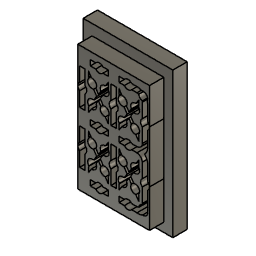
Case v4 (Autodesk Fusion 360 design; units mm, degrees)
Autodesk Fusion 360 part; units mm, degrees
note: some values were not read from the file. Set by a fixed rule: which sketch regions a step uses.
sketch "Skizze1" plane through (0, 0, 0) normal (0, 1, 0) x (1, 0, 0)
  line L0 (0, 0) -> (50, 0)
  line L1 (50, 0) -> (50, -81)
  line L2 (50, -81) -> (0, -81)
  line L3 (0, -81) -> (0, 0)
  line L4 (5, 0) -> (5, -5)
  line L5 (5, -5) -> (5, -75)
  line L6 (5, -75) -> (45, -75)
  line L7 (45, -75) -> (45, -5)
  line L8 (5, -5) -> (45, -5)
  line L9 (12, -10) -> (22, -10)
  line L10 (22, -10) -> (22, -13)
  line L11 (22, -13) -> (12, -13)
  line L12 (12, -13) -> (12, -10)
  line L13 (28, -10) -> (38, -10)
  line L14 (38, -10) -> (38, -13)
  line L15 (38, -13) -> (28, -13)
  line L16 (28, -13) -> (28, -10)
  line L17 (9, -16) -> (6, -16)
  line L18 (6, -16) -> (6, -36)
  line L19 (6, -36) -> (9, -36)
  line L20 (9, -36) -> (9, -16)
  line L21 (23.5, -16) -> (26.5, -16)
  line L22 (26.5, -16) -> (26.5, -36)
  line L23 (26.5, -36) -> (23.5, -36)
  line L24 (23.5, -36) -> (23.5, -16)
  line L25 (41, -16) -> (44, -16)
  line L26 (44, -16) -> (44, -36)
  line L27 (44, -36) -> (41, -36)
  line L28 (41, -36) -> (41, -16)
  line L29 (38, -42) -> (28, -42)
  line L30 (22, -39) -> (22, -42)
  line L31 (38, -39) -> (38, -42)
  line L32 (12, -39) -> (22, -39)
  line L33 (28, -39) -> (38, -39)
  line L34 (22, -42) -> (12, -42)
  line L35 (28, -42) -> (28, -39)
  line L36 (12, -42) -> (12, -39)
  line L37 (23.5, -45) -> (26.5, -45)
  line L38 (28, -68) -> (38, -68)
  line L39 (6, -45) -> (6, -65)
  line L40 (44, -65) -> (41, -65)
  line L41 (9, -65) -> (9, -45)
  line L42 (26.5, -45) -> (26.5, -65)
  line L43 (38, -71) -> (28, -71)
  line L44 (26.5, -65) -> (23.5, -65)
  line L45 (41, -45) -> (44, -45)
  line L46 (41, -65) -> (41, -45)
  line L47 (23.5, -65) -> (23.5, -45)
  line L48 (12, -68) -> (22, -68)
  line L49 (12, -71) -> (12, -68)
  line L50 (38, -68) -> (38, -71)
  line L51 (9, -45) -> (6, -45)
  line L52 (22, -71) -> (12, -71)
  line L53 (28, -71) -> (28, -68)
  line L54 (44, -45) -> (44, -65)
  line L55 (6, -65) -> (9, -65)
  line L56 (22, -68) -> (22, -71)
  line L57 (11, -65) -> (11, -62)
  line L58 (22, -45) -> (22, -48)
  line L59 (22, -48) -> (11, -65)
  line L60 (11, -62) -> (22, -45)
  line L61 (22, -65) -> (22, -62)
  line L62 (22, -62) -> (11, -45)
  line L63 (11, -45) -> (11, -48)
  line L64 (11, -48) -> (22, -65)
  line L65 (22, -16) -> (22, -19)
  line L66 (22, -19) -> (11, -36)
  line L67 (11, -36) -> (11, -33)
  line L68 (11, -19) -> (22, -36)
  line L69 (11, -16) -> (11, -19)
  line L70 (11, -33) -> (22, -16)
  line L71 (22, -36) -> (22, -33)
  line L72 (22, -33) -> (11, -16)
  line L73 (22, -45) -> (22, -48)
  line L74 (22, -48) -> (11, -65)
  line L75 (11, -65) -> (11, -62)
  line L76 (11, -48) -> (22, -65)
  line L77 (11, -45) -> (11, -48)
  line L78 (11, -62) -> (22, -45)
  line L79 (22, -65) -> (22, -62)
  line L80 (22, -62) -> (11, -45)
  line L81 (39, -16) -> (39, -19)
  line L82 (39, -19) -> (28, -36)
  line L83 (28, -36) -> (28, -33)
  line L84 (28, -19) -> (39, -36)
  line L85 (28, -16) -> (28, -19)
  line L86 (28, -33) -> (39, -16)
  line L87 (39, -36) -> (39, -33)
  line L88 (39, -33) -> (28, -16)
  arc A0 (44, -45) -> (38, -39) centre (38.387, -44.613) ccw
  arc A1 (38, -42) -> (44, -36) centre (38.3769, -36.3769) ccw
  arc A2 (38, -39) -> (41, -36) centre (37.7778, -35.7778) ccw
  arc A3 (38, -68) -> (41, -65) centre (38, -65) ccw
  arc A4 (38, -71) -> (44, -65) centre (38, -65) ccw
  arc A5 (41, -16) -> (38, -13) centre (38, -16) ccw
  arc A6 (44, -16) -> (38, -10) centre (38.75, -15.25) ccw
  line L89 (28, -65) -> (28, -62)
  line L90 (39, -62) -> (28, -45)
  line L91 (28, -65) -> (28, -62)
  line L92 (39, -45) -> (39, -48)
  line L93 (39, -65) -> (39, -62)
  line L94 (28, -62) -> (39, -45)
  line L95 (28, -45) -> (28, -48)
  line L96 (39, -48) -> (28, -65)
  line L97 (39, -48) -> (28, -65)
  line L98 (28, -62) -> (39, -45)
  line L99 (39, -65) -> (39, -62)
  line L100 (28, -45) -> (28, -48)
  line L101 (39, -62) -> (28, -45)
  line L102 (39, -45) -> (39, -48)
  line L103 (28, -48) -> (39, -65)
  line L104 (28, -48) -> (39, -65)
  arc A7 (41, -45) -> (38, -42) centre (38, -45) ccw
  point P0 (21.5707, -67.1048)
  dimension "d1" = 50
  dimension "d2" = 81
  dimension "d3" = 10
  dimension "d4" = 10
  dimension "d5" = 3
  dimension "d6" = 20
  dimension "d7" = 3
  dimension "d8" = 20
  dimension "d9" = 3
  dimension "d10" = 20
  dimension "d11" = 10
  dimension "d12" = 10
  dimension "d13" = 3
  dimension "d14" = 20
  dimension "d15" = 3
  dimension "d16" = 20
  dimension "d17" = 3
  dimension "d18" = 20
  dimension "d19" = 10
  dimension "d20" = 10
  dimension "d25" = 70
  constraint horizontal L0
  constraint vertical L1
  constraint horizontal L2
  constraint vertical L3
  constraint coincident L0.start L3.end
  constraint coincident L0 L4.start
  constraint perpendicular L0 L4
  constraint perpendicular L0 L5
  constraint perpendicular L5 L6
  constraint perpendicular L6 L7
  constraint perpendicular L7 L8
  constraint horizontal L9
  constraint vertical L10
  constraint horizontal L11
  constraint vertical L12
  constraint horizontal L13
  constraint vertical L14
  constraint horizontal L15
  constraint vertical L16
  constraint horizontal L17
  constraint vertical L18
  constraint horizontal L19
  constraint vertical L20
  constraint horizontal L21
  constraint vertical L22
  constraint horizontal L23
  constraint vertical L24
  constraint horizontal L25
  constraint vertical L26
  constraint horizontal L27
  constraint vertical L28
  constraint horizontal L32
  constraint vertical L30
  constraint horizontal L34
  constraint vertical L36
  constraint horizontal L33
  constraint vertical L31
  constraint horizontal L29
  constraint vertical L35
  constraint horizontal L51
  constraint vertical L39
  constraint horizontal L55
  constraint vertical L41
  constraint horizontal L37
  constraint vertical L42
  constraint horizontal L44
  constraint vertical L47
  constraint horizontal L45
  constraint vertical L54
  constraint horizontal L40
  constraint vertical L46
  constraint horizontal L48
  constraint vertical L56
  constraint horizontal L52
  constraint vertical L49
  constraint horizontal L38
  constraint vertical L50
  constraint horizontal L43
  constraint vertical L53
  constraint vertical L57
  constraint parallel L47 L58
  constraint parallel L59 L60
  constraint parallel L58 L61
  constraint parallel L61 L63
  constraint parallel L62 L64
  constraint vertical L67
  constraint parallel L66 L70
  constraint parallel L65 L71
  constraint parallel L69 L71
  constraint parallel L68 L72
  constraint vertical L75
  constraint parallel L74 L78
  constraint parallel L73 L79
  constraint parallel L77 L79
  constraint parallel L76 L80
  constraint vertical L83
  constraint parallel L82 L86
  constraint parallel L81 L87
  constraint parallel L85 L87
  constraint parallel L84 L88
  constraint tangent A0 A2
  constraint tangent L46 A3
  constraint tangent L54 A4
  constraint tangent L28 A5
  constraint vertical L89
  constraint parallel L94 L96
  constraint parallel L99 L102
  constraint parallel L95 L99
  constraint parallel L101 L104
  constraint vertical L91
  constraint parallel L97 L98
  constraint parallel L92 L93
  constraint parallel L93 L100
  constraint parallel L90 L103
  constraint tangent L46 A7
  measures "d1" distance of L0.start L0.end
  measures "d2" distance of L0.start L2.end
  measures "d3" distance of L10.end L11.end
  measures "d4" distance of L14.end L15.end
  measures "d5" distance of L17.start L17.end
  measures "d6" distance of L17.start L19.end
  measures "d7" distance of L21.start L21.end
  measures "d8" distance of L21.start L23.end
  measures "d9" distance of L25.start L25.end
  measures "d10" distance of L25.start L27.end
  measures "d11" distance of L30.end L34.end
  measures "d12" distance of L29.start L29.end
  measures "d13" distance of L41.end L39.start
  measures "d14" distance of L41.end L41.start
  measures "d15" distance of L37.end L37.start
  measures "d16" distance of L37.start L44.end
  measures "d17" distance of L45.start L45.end
  measures "d18" distance of L45.start L40.end
  measures "d19" distance of L52.start L49.start
  measures "d20" distance of L43.end L43.start
  measures "d25" distance of L4.end L5.end
extrude "Extrusion1" add sketch "Skizze1" along normal blind 8 contours L0 L1 L2 L3
extrude "Extrusion2" add sketch "Skizze1" along normal blind 4 contours L5 L6 L7 L8
sketch "Skizze2" plane through (0, 0, 0) normal (0, 1, 0) x (1, 0, 0)
  circle A0 centre (20, -60) radius 2.5
  circle A1 centre (13, -60) radius 2.5
  circle A2 centre (30, -60) radius 2.5
  circle A3 centre (37, -60) radius 2.5
  circle A4 centre (25, -55) radius 2.5
  circle A5 centre (7.5, -55) radius 2.5
  circle A6 centre (42.5, -55) radius 2.5
  circle A7 centre (17, -69.5) radius 2.5
  circle A8 centre (33, -69.5) radius 2.5
  circle A9 centre (41.5, -68) radius 2.5
  circle A10 centre (33, -69.5) radius 2.5
  circle A11 centre (42, -43) radius 1.5
  circle A12 centre (39.5, -40.5) radius 1.5
  circle A13 centre (33, -40.5) radius 2.5
  circle A14 centre (42.5, -26) radius 2.5
  circle A15 centre (33, -11.5) radius 2.5
  circle A16 centre (7.5, -26) radius 2.5
  circle A17 centre (17, -40.5) radius 2.5
  circle A18 centre (25, -26) radius 2.5
  circle A19 centre (17, -11.5) radius 2.5
  circle A20 centre (13, -31) radius 2.5
  circle A21 centre (30, -31) radius 2.5
  circle A22 centre (20, -31) radius 2.5
  circle A23 centre (37, -31) radius 2.5
  circle A24 centre (42, -38) radius 1.5
  line L0 (28, -62) -> (28, -45)
  line L1 (28, -45) -> (39, -45)
  line L2 (41, -65) -> (41.5, -65)
  line L3 (41.5, -65) -> (41.5, -68)
  line L4 (39, -62) -> (39, -60)
  line L5 (37, -60) -> (39, -60)
  line L6 (41, -16) -> (41.5, -16)
  line L7 (41.5, -16) -> (41.5, -13)
  circle A25 centre (41.5, -13) radius 2.5
  circle A26 centre (13, -50) radius 2.5
  circle A27 centre (20, -50) radius 2.5
  circle A28 centre (37, -50) radius 2.5
  circle A29 centre (30, -50) radius 2.5
  circle A30 centre (13, -21) radius 2.5
  circle A31 centre (20, -21) radius 2.5
  circle A32 centre (30, -21) radius 2.5
  circle A33 centre (37, -21) radius 2.5
  dimension "d30" = 5
  dimension "d31" = 5
  dimension "d32" = 5
  dimension "d33" = 5
  dimension "d34" = 5
  dimension "d35" = 5
  dimension "d36" = 5
  dimension "d37" = 5
  dimension "d38" = 5
  dimension "d39" = 5
  dimension "d40" = 3
  dimension "d41" = 3
  dimension "d42" = 5
  dimension "d43" = 5
  dimension "d44" = 5
  dimension "d45" = 5
  dimension "d46" = 5
  dimension "d47" = 5
  dimension "d48" = 5
  dimension "d49" = 5
  dimension "d50" = 5
  dimension "d51" = 5
  dimension "d52" = 3
  dimension "d57" = 17
  dimension "d58" = 11
  dimension "d59" = 0.5
  dimension "d60" = 3
  dimension "d61" = 2
  dimension "d62" = 2
  dimension "d63" = 0.5
  dimension "d64" = 3
  dimension "d65" = 5
  constraint vertical L0
  constraint perpendicular L0 L1
  constraint horizontal L2
  constraint perpendicular L2 L3
  constraint coincident A9.centre L3.end
  constraint vertical L4
  constraint coincident A3.centre L5.start
  constraint horizontal L6
  constraint perpendicular L6 L7
  constraint coincident L7.end A25.centre
  measures "d30" diameter of A0
  measures "d31" diameter of A1
  measures "d32" diameter of A2
  measures "d33" diameter of A3
  measures "d34" diameter of A4
  measures "d35" diameter of A6
  measures "d36" diameter of A7
  measures "d37" diameter of A8
  measures "d38" diameter of A9
  measures "d39" diameter of A10
  measures "d40" diameter of A11
  measures "d41" diameter of A12
  measures "d42" diameter of A14
  measures "d43" diameter of A15
  measures "d44" diameter of A16
  measures "d45" diameter of A17
  measures "d46" diameter of A18
  measures "d47" diameter of A19
  measures "d48" diameter of A20
  measures "d49" diameter of A21
  measures "d50" diameter of A22
  measures "d51" diameter of A23
  measures "d52" diameter of A24
  measures "d57" distance of L0.start L0.end
  measures "d58" distance of L0.end L1.end
  measures "d59" distance of L2.start L2.end
  measures "d60" distance of L2.end A9.centre
  measures "d61" distance of L4.start L4.end
  measures "d62" distance of L4.end A3.centre
  measures "d63" distance of L6.start L6.end
  measures "d64" distance of L6.end L7.end
  measures "d65" diameter of A25
extrude "Extrusion3" add sketch "Skizze1" against normal blind 8 contours L5 L6 L7 L8
extrude "Extrusion4" cut sketch "Skizze2" against normal blind 8
